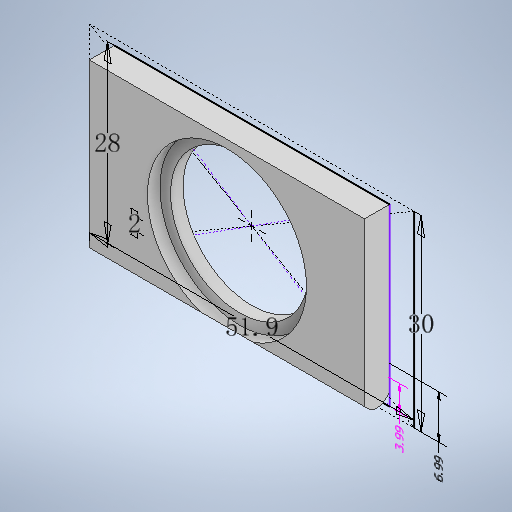
# Autodesk Inventor part: 可调平台
Saved by Autodesk Inventor 2025 (Build 290162000, 162)
## iProperties
Created: 2024-08-28
Part Number: 可调平台
Material: 常规
Document SubType Name: Sheet Metal
Designer: Leexi
Density: 1 g/cm^3
Sheet Metal Rule: 默认_mm
Appearance: 默认
Author: Leexi
Autodesk Inventor part; units mm, degrees
ref_plane "YZ Plane" through (0, 0, 0) normal (1, 0, 0) x (0, 1, 0)
ref_plane "XZ Plane" through (0, 0, 0) normal (0, 1, 0) x (-1, 0, 0)
ref_plane "XY Plane" through (0, 0, 0) normal (0, 0, 1) x (1, 0, 0)
sketch "草图1" plane through (0, 0, 0) normal (0, 0, 1) x (1, 0, 0)
  line L0 (-25.95, -15) -> (25.95, -15) construction
  line L1 (25.95, -15) -> (25.95, 15)
  line L2 (25.95, 15) -> (-25.95, 15) construction
  line L3 (-25.95, 15) -> (-25.95, -15) construction
  line L4 (-25.95, -15) -> (25.95, 15) construction
  line L5 (25.95, -15) -> (-25.95, 15) construction
  line L6 (0, 0) -> (-17.3154, 10.0089) construction
  line L7 (0, 0) -> (17.3154, 10.0089) construction
  line L8 (22, -14) -> (-22, -14)
  line L9 (-22, -14) -> (-22, 14)
  line L10 (-22, 14) -> (22, 14)
  line L11 (22, 14) -> (22, -14)
  line L12 (22, -14) -> (-22, 14) construction
  line L13 (-22, -14) -> (22, 14) construction
  line L14 (0, 0) -> (17.3154, -10.0089) construction
  line L15 (-17.3154, -10.0089) -> (-17.3154, -8.0089) construction
  point P0 (17.3154, -8.0089)
  point P1 (17.3154, -8.0089)
  dimension "d0" = 51.9
  dimension "d1" = 30
  dimension "d6" = 28
  dimension "d27" = 2
  constraints: 32 end point, 5 coincident, 4 midpoint, 4 parallel, 3 point on line, 2 horizontal, 2 perpendicular, 1 vertical, 4 other
  measures "d0" distance of L0.start L0.end
  measures "d1" distance of L1.end L0.end
  measures "d6" distance of L8.end L9.end
  measures "d27" distance of L15.start L15.end
extrude "拉伸1" add sketch "草图1" along normal blind 4
hole "孔1" at (17.3154, 10.0089, 0) at (-17.3154, 10.0089, 0) at (17.3154, -8.0089, 0) at (-17.3154, -8.0089, 0) direction (0, 0, 1) diameter 4.95 depth 2.5 tip angle 118
sketch "草图2" plane through (0, 0, 4) normal (0, 0, 1) x (1, 0, 0)
  point P0 (0, 0)
  point P1 (0, 0)
  constraints: 1 coincident
hole "孔2" at (0, 0, 4) direction (0, 0, -1) diameter 22 end through all counterbore diameter 25.4 counterbore depth 2
chamfer "倒角1" distance 2 angle 45 2 edges at (0, -14, 0) (0, -14, 4)
fillet "圆角1" radius 2 1 edges at (0, -14, 2)
equation "\"d21\" = 厚度"
equation "\"折弯半径\" = 厚度"
equation "\"折弯释压宽度\" = 厚度"
equation "\"折弯释压深度\" = 0.5 * 厚度"
equation "\"拐角释压尺寸\" = 4 * 厚度"
equation "\"最小余量\" = 2 * 厚度"
equation "\"过渡半径\" = 折弯半径"
equation "\"Jacobi半径尺寸\" = 折弯半径"
equation "\"厚度\" = 0.5"
